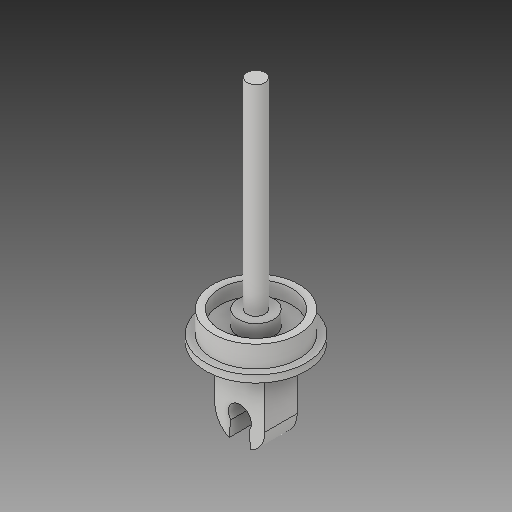
# Autodesk Inventor part: Bottom
Saved by Autodesk Inventor 2019 (Build 230136000, 136)
## iProperties
Created: 2019-03-03
Part Number: Bottom
Material: Generic
Document SubType Name: Modeling
Designer: alarr
Density: 1 g/cm^3
Appearance: Default
Author: alarr
Autodesk Inventor part; units mm, degrees
ref_plane "YZ Plane" through (0, 0, 0) normal (1, 0, 0) x (0, 1, 0)
ref_plane "XZ Plane" through (0, 0, 0) normal (0, 1, 0) x (-1, 0, 0)
ref_plane "XY Plane" through (0, 0, 0) normal (0, 0, 1) x (1, 0, 0)
sketch "Sketch1" plane through (0, 0, 0) normal (0, 0, 1) x (1, 0, 0)
  arc A0 (-4.445, 0) -> (4.445, 0) centre (0, 0) ccw
  line L0 (-4.445, 0) -> (-4.445, 8.89)
  line L1 (-4.445, 8.89) -> (4.445, 8.89)
  line L2 (4.445, 8.89) -> (4.445, 0)
  arc A1 (4.445, 0) -> (-4.445, 0) centre (0, 0) ccw construction
  dimension "d0" = 8.89
  dimension "d1" = 8.89
  constraints: 6 end point, 4 point on circle, 2 centre point, 2 tangent, 1 coincident, 1 perpendicular, 1 vertical
  measures "d0" distance between parallel lines of L2 L0
  measures "d1" distance of L1.end L2.end
sketch "Sketch1 outline for Extrusion1" plane through (0, 0, 0) normal (0, 0, 1) x (1, 0, 0)
  line L0 (-4.445, 8.89) -> (-4.445, 0)
  line L1 (4.445, 8.89) -> (-4.445, 8.89)
  line L2 (4.445, 0) -> (4.445, 8.89)
  arc A0 (-4.445, 0) -> (4.445, 0) centre (0, 0) ccw
extrude "Extrusion1" add sketch "Sketch1 outline for Extrusion1" along normal mid plane 5.715
sketch "Sketch2" plane through (0, 0, 2.8575) normal (0, 0, 1) x (1, 0, 0)
  arc A0 (1.651, -1.184577) -> (-1.651, -1.184577) centre (0, 0) ccw
  line L0 (1.651, -1.184577) -> (1.905, -4.016093)
  line L1 (0, 0) -> (0, -4.445) construction
  line L2 (-1.651, -1.184577) -> (-1.905, -4.016093)
  arc A1 (0, -2.032) -> (1.651, -1.184577) centre (0, 0) ccw construction
  arc A2 (-1.651, -1.184577) -> (0, -2.032) centre (0, 0) ccw construction
  arc A3 (-4.445, 0) -> (4.445, 0) centre (0, 0) ccw
  dimension "d4" = 4.064
  dimension "d5" = 3.81
  dimension "d6" = 3.302
  constraints: 8 point on circle, 6 end point, 3 centre point, 2 symmetric about line, 1 coincident, 1 point on line
  measures "d4" diameter of A0
  measures "d5" distance of L0.end L2.end
  measures "d6" distance of L0.start L2.start
sketch "Sketch2 outline for Extrusion2" plane through (0, 0, 2.8575) normal (0, 0, 1) x (1, 0, 0)
  line L0 (1.905, -4.016093) -> (1.651, -1.184577)
  arc A0 (-1.905, -4.016093) -> (1.905, -4.016093) centre (0, 0) ccw
  line L1 (-1.651, -1.184577) -> (-1.905, -4.016093)
  arc A1 (1.651, -1.184577) -> (-1.651, -1.184577) centre (0, 0) ccw
extrude "Extrusion2" cut sketch "Sketch2 outline for Extrusion2" against normal through all
sketch "Sketch3" plane through (0, 0, 0) normal (0, 0, 1) x (1, 0, 0)
  line L0 (4.445, 8.89) -> (-4.445, 8.89)
  line L1 (0, 7.62) -> (4.445, 8.89)
  line L2 (4.445, 8.89) -> (8.89, 10.16)
  line L3 (8.89, 10.16) -> (8.89, 11.43)
  line L4 (8.89, 11.43) -> (7.62, 11.43)
  line L5 (7.62, 11.43) -> (7.62, 15.24)
  line L6 (7.62, 15.24) -> (0, 15.24)
  line L7 (0, 15.24) -> (0, 7.62)
  line L8 (0, 0) -> (0, 8.89) construction
  line L9 (0, -7.867311) -> (0, 19.091219)
  dimension "d9" = 8.89
  dimension "d10" = 6.35
  dimension "d11" = 3.81
  dimension "d12" = 1.27
  dimension "d13" = 1.27
  constraints: 16 end point, 5 perpendicular, 1 collinear, 1 midpoint, 1 point on line
  measures "d9" distance between parallel lines of L3 L7
  measures "d10" distance between parallel lines of L6 L0
  measures "d11" distance of L4.end L5.end
  measures "d12" distance of L3.end L4.end
  measures "d13" distance of L1.start L8.end
sketch "Sketch3 outline for Revolution1" plane through (0, 0, 0) normal (0, 0, 1) x (1, 0, 0)
  line L0 (0, 15.24) -> (0, 7.62)
  line L1 (7.62, 15.24) -> (0, 15.24)
  line L2 (7.62, 11.43) -> (7.62, 15.24)
  line L3 (8.89, 11.43) -> (7.62, 11.43)
  line L4 (8.89, 10.16) -> (8.89, 11.43)
  line L5 (4.445, 8.89) -> (8.89, 10.16)
  line L6 (0, 7.62) -> (4.445, 8.89)
revolve "Revolution1" add sketch "Sketch3 outline for Revolution1" angle 360 about axis through (0, -10, 0) along (0, 1, 0)
sketch "Sketch4" plane through (0, 15.24, 0) normal (0, 1, 0) x (1, 0, 0)
  circle A0 centre (0, 0) radius 3.175
  circle A1 centre (0, 0) radius 7.62 projected
  circle A2 centre (0, 0) radius 6.35
  dimension "d15" = 6.35
  dimension "d16" = 1.27
  constraints: 2 centre point, 1 coincident
  measures "d15" diameter of A0
  measures "d16" radial gap between concentric circles of A1 A2
sketch "Sketch4 outline for Extrusion3" plane through (0, 15.24, 0) normal (0, 1, 0) x (1, 0, 0)
  circle A0 centre (0, 0) radius 6.35
  circle A1 centre (0, 0) radius 3.175
extrude "Extrusion3" cut sketch "Sketch4 outline for Extrusion3" against normal blind 2.54
sketch "Sketch5" plane through (0, 15.24, 0) normal (0, 1, 0) x (1, 0, 0)
  circle A0 centre (0, 0) radius 1.5875
  dimension "d19" = 3.175
  constraints: 1 centre point, 1 coincident
  measures "d19" diameter of A0
sketch "Sketch5 outline for Extrusion4" plane through (0, 15.24, 0) normal (0, 1, 0) x (1, 0, 0)
  circle A0 centre (0, 0) radius 1.5875
extrude "Extrusion4" add sketch "Sketch5 outline for Extrusion4" along normal blind 35.56
body "Solid1"
